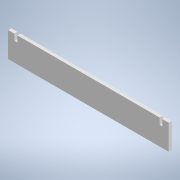
# Autodesk Inventor part: BackBrace
Saved by Autodesk Inventor 2020 (Build 240168000, 168)
## iProperties
Created: 2019-08-12
Part Number: BackBrace
Material: Generic
Document SubType Name: Modeling
Designer: eugen
Density: 1 g/cm^3
Appearance: Default
Author: eugen
Autodesk Inventor part; units mm, degrees
ref_plane "YZ Plane" through (0, 0, 0) normal (1, 0, 0) x (0, 1, 0)
ref_plane "XZ Plane" through (0, 0, 0) normal (0, 1, 0) x (-1, 0, 0)
ref_plane "XY Plane" through (0, 0, 0) normal (0, 0, 1) x (1, 0, 0)
sketch "Sketch1" plane through (0, 0, 0) normal (0, 0, 1) x (1, 0, 0)
  line L0 (0, 0) -> (324.7199, 0)
  line L1 (324.7199, 0) -> (324.7199, 50.8)
  line L2 (324.7199, 50.8) -> (0, 50.8)
  line L3 (0, 50.8) -> (0, 0)
  line L4 (12.7, 50.8) -> (18.542, 50.8)
  line L5 (18.542, 50.8) -> (18.542, 39.37)
  line L6 (17.272, 38.1) -> (13.97, 38.1)
  line L7 (12.7, 39.37) -> (12.7, 50.8)
  line L8 (306.178, 50.8) -> (312.0199, 50.8)
  line L9 (312.0199, 50.8) -> (312.0199, 39.37)
  line L10 (310.75, 38.1) -> (307.4479, 38.1)
  line L11 (306.1779, 39.37) -> (306.178, 50.8)
  arc A0 (12.7, 39.37) -> (13.97, 38.1) centre (13.97, 39.37) ccw
  arc A1 (17.272, 38.1) -> (18.542, 39.37) centre (17.272, 39.37) ccw
  arc A2 (306.1779, 39.37) -> (307.4479, 38.1) centre (307.4479, 39.37) ccw
  arc A3 (310.75, 38.1) -> (312.0199, 39.37) centre (310.75, 39.37) ccw
  point P0 (18.542, 38.1)
  point P1 (12.7, 38.1)
  point P2 (312.0199, 38.1)
  point P3 (306.178, 38.1)
  dimension "d0" = 324.7199
  dimension "d1" = 50.8
  dimension "d2" = 12.7
  dimension "d3" = 12.7
  dimension "d4" = 5.842
  dimension "d5" = 12.7
  dimension "d8" = 1.27
  constraints: 24 end point, 10 point on line, 8 point on circle, 8 tangent, 6 parallel, 4 centre point, 3 equal radius, 3 horizontal, 3 perpendicular, 2 collinear
  measures "d0" distance of L1.end L2.end
  measures "d1" distance of L0.end L1.end
  measures "d2" distance between parallel lines of L3 L7
  measures "d3" distance between parallel lines of L1 L9
  measures "d4" distance between parallel lines of L5 L7
  measures "d5" distance of L4.end point (18.542, 38.1)
  measures "d8" radius of A0
extrude "Extrusion1" add sketch "Sketch1" along normal blind 6.35 contours L3 L2 L7 A0 L6 A1 L5 L11 A2 L10 A3 L9 L1 L0
body "Solid1"
